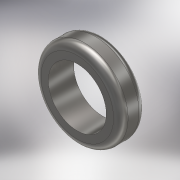
# Autodesk Inventor part: MF128ZZ
Saved by Autodesk Inventor 2018.2 (Build 222227000, 227)
## iProperties
Created: 2017-12-11
Part Number: MF128ZZ
Material: ステンレス鋼
Document SubType Name: Modeling
Designer: kuwano
Density: 8 g/cm^3
Appearance: 半つや出し
Mass: 1.63467 g
Surface Area: 3.12324 cm^2
Volume: 0.204333 cm^3
Author: kuwano
Autodesk Inventor part; units mm, degrees
ref_plane "YZ Plane" through (0, 0, 0) normal (1, 0, 0) x (0, 1, 0)
ref_plane "XZ Plane" through (0, 0, 0) normal (0, 1, 0) x (-1, 0, 0)
ref_plane "XY Plane" through (0, 0, 0) normal (0, 0, 1) x (1, 0, 0)
sketch "スケッチ1" plane through (0, 0, 0) normal (0, 1, 0) x (-1, 0, 0)
  circle A0 centre (0, 0) radius 6
  circle A1 centre (0, 0) radius 4
  dimension "d0" = 12
  dimension "d1" = 8
  constraints: 2 centre point, 2 coincident
  measures "d0" diameter of A0
  measures "d1" diameter of A1
extrude "押し出し1" add sketch "スケッチ1" along normal mid plane 3.5
fillet "フィレット1" radius 1 2 edges at (6, 1.75, 0) (6, -1.75, 0)
